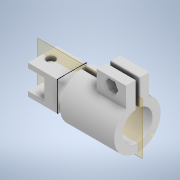
# Autodesk Inventor part: Arm connection
Saved by Autodesk Inventor 2021 (Build 250183000, 183)
## iProperties
Created: 2021-04-09
Part Number: Arm connection
Material: Generic
Document SubType Name: Modeling
Designer: Olivi
Density: 1 g/cm^3
Appearance: Default
Author: Olivi
Autodesk Inventor part; units mm, degrees
ref_plane "YZ Plane" through (0, 0, 0) normal (1, 0, 0) x (0, 1, 0)
sketch "Sketch1" plane through (0, 0, 0) normal (0, 0, 1) x (1, 0, 0)
  line L0 (0, 0) -> (0, 2.5)
  line L1 (0, 2.5) -> (8.5, 2.5)
  line L2 (8.5, 2.5) -> (8.5, 12.7)
  line L3 (8.5, 12.7) -> (0, 12.7)
  line L4 (0, 12.7) -> (0, 15.2)
  line L5 (0, 15.2) -> (15, 15.2)
  line L6 (15, 15.2) -> (15, 0)
  line L7 (15, 0) -> (0, 0)
  dimension "d0" = 2.5
  dimension "d1" = 8.5
  dimension "d2" = 10.2
  dimension "d3" = 2.5
  dimension "d4" = 15
  constraints: 16 end point, 6 perpendicular, 1 horizontal, 1 vertical
  measures "d0" distance of L0.start L0.end
  measures "d1" distance of L0.end L1.end
  measures "d2" distance of L1.end L2.end
  measures "d3" distance of L3.end L4.end
  measures "d4" distance of L4.end L5.end
extrude "Extrusion1" add sketch "Sketch1" along normal blind 15
ref_plane "Work Plane1" through (18, 0, 0) normal (1, 0, 0) x (0, 0, -1)
sketch "Sketch3" plane through (15, 0, 0) normal (1, 0, 0) x (0, 0, -1)
  line L0 (0, 15.2) -> (-15, 15.2) projected
  line L1 (-15, 15.2) -> (0, 15.2)
  line L2 (0, 0) -> (-15, 0) projected
  line L3 (0, 15.2) -> (0, 0)
  line L4 (-15, 2.5) -> (-15, 0) projected
  line L5 (0, 0) -> (-15, 0)
  line L6 (-15, 15.2) -> (-15, 12.7) projected
  line L7 (-15, 0) -> (-15, 15.2)
  constraints: 8 end point, 3 perpendicular, 1 horizontal
sketch "Sketch4" plane through (18, 0, 0) normal (1, 0, 0) x (0, 0, -1)
  circle A0 centre (-7.5, 7.7) radius 9
  line L0 (0, 15.2) -> (-15, 15.2) projected
  line L1 (-15, 0) -> (-15, 15.2) projected
  point P0 (0, 0)
  dimension "d10" = 18
  dimension "d11" = 7.5
  dimension "d12" = 7.5
  constraints: 1 centre point
  measures "d10" diameter of A0
  measures "d11" distance from line of L0 A0.centre
  measures "d12" distance from line of L1 A0.centre
ref_plane "Work Plane2" through (21, 7.7, 7.5) normal (1, 0, 0) x (0, 0, -1)
sketch "Sketch5" plane through (21, 7.7, 7.5) normal (1, 0, 0) x (0, 0, -1)
  circle A0 centre (0, 0) radius 12
  point P0 (7.5, -7.7)
  dimension "d18" = 24
  constraints: 1 centre point
  measures "d18" diameter of A0
sketch "Sketch4 outline for Loft2" plane through (18, 0, 0) normal (1, 0, 0) x (0, 0, -1)
  circle A0 centre (-7.5, 7.7) radius 9
sketch "Sketch5 outline for Loft2" plane through (21, 7.7, 7.5) normal (1, 0, 0) x (0, 0, -1)
  circle A0 centre (0, 0) radius 12
loft "Loft2" add profiles "Sketch4 outline for Loft2", "Sketch5 outline for Loft2" section 1 edges at (15, 7.6, 0) (15, 15.2, 7.5) (15, 7.6, 15) (15, 0, 7.5)
sketch "Sketch6" plane through (21, 7.7, 7.5) normal (1, 0, 0) x (0, 0, -1)
  circle A0 centre (0, 0) radius 7.75
  circle A1 centre (0, 0) radius 12
  point P0 (7.5, -7.7)
  dimension "d25" = 15.5
  constraints: 2 centre point, 1 coincident
  measures "d25" diameter of A0
extrude "Extrusion2" add sketch "Sketch6" along normal blind 28
ref_plane "Work Plane3" through (0, 0, 7.5) normal (0, 0, 1) x (1, 0, 0)
sketch "Sketch7" plane through (0, 0, 7.5) normal (0, 0, 1) x (1, 0, 0)
  line L0 (21, 19.7) -> (49, 19.7)
  line L1 (49, 19.7) -> (21, 19.7)
  line L2 (21, 16.241288) -> (21, -0.841288)
  line L3 (21, 15.217594) -> (49, 15.217594)
  line L4 (49, -4.3) -> (49, 19.7)
  line L5 (49, 15.217594) -> (49, 19.7)
  line L6 (21, 19.7) -> (21, 16.241288)
  line L7 (21, 19.7) -> (21, 15.217594)
  point P0 (0, 0)
  constraints: 8 end point, 3 point on line, 2 collinear, 1 perpendicular
extrude "Extrusion3" cut sketch "Sketch7" against normal mid plane 2
sketch "Sketch8" plane through (49, 7.7, 7.5) normal (1, 0, 0) x (0, 0, -1)
  point P0 (7.5, -7.7)
sketch "Sketch10" plane through (49, 7.7, 7.5) normal (1, 0, 0) x (0, 0, -1)
  arc A0 (-1, 11.958261) -> (-8.428903, 8.541288) centre (0, 0) ccw
  line L0 (-1, 11.958261) -> (-1, 20.958261)
  line L1 (-1, 20.958261) -> (-6, 20.958261)
  line L2 (-6, 20.958261) -> (-6, 10.392305)
  arc A1 (8.428903, 8.541288) -> (1, 11.958261) centre (0, 0) ccw
  line L3 (1, 11.958261) -> (1, 20.958261)
  line L4 (1, 20.958261) -> (6, 20.958261)
  line L5 (6, 20.958261) -> (6, 10.392305)
  arc A2 (-1, 11.958261) -> (-6, 10.392305) centre (0, 0) ccw
  line L6 (1, 7.685213) -> (1, 11.958261)
  arc A3 (6, 10.392305) -> (1, 11.958261) centre (0, 0) ccw
  point P0 (7.5, -7.7)
  dimension "d33" = 9
  dimension "d34" = 5
  dimension "d35" = 5
  constraints: 12 end point, 6 point on circle, 3 perpendicular, 2 centre point, 2 point on line, 1 concentric, 1 parallel, 1 vertical
  measures "d33" distance of L0.start L0.end
  measures "d34" distance of L0.end L1.end
  measures "d35" distance of L3.end L4.end
extrude "Extrusion4" add sketch "Sketch10" against normal blind 15
sketch "Sketch11" plane through (49, 18.092305, 1.5) normal (0, 0, -1) x (-1, 0, 0)
  circle A0 centre (7.5, 6.35) radius 1.75
  point P0 (49, -18.092305)
  dimension "d38" = 3.5
  constraints: 1 centre point
  measures "d38" diameter of A0
extrude "Extrusion5" cut sketch "Sketch11" against normal through all
sketch "Sketch12" plane through (49, 18.092305, 1.5) normal (0, 0, -1) x (-1, 0, 0)
  circle A0 centre (7.5, 6.35) radius 1.75 projected
  circle A1 centre (7.5, 6.35) radius 3
  point P0 (49, -18.092305)
  dimension "d41" = 6
  constraints: 1 centre point, 1 coincident
  measures "d41" diameter of A1
extrude "Extrusion6" cut sketch "Sketch12" against normal blind 2.5 contours A0 | A1
sketch "Sketch13" plane through (0, 0, 8.5) normal (0, 0, -1) x (-1, 0, 0)
  point P0 (0, 0)
sketch "Sketch14" plane through (49, 18.092305, 13.5) normal (0, 0, 1) x (1, 0, 0)
  circle A0 centre (-7.5, 6.35) radius 1.75
  line L0 (-3.920428, 6.35) -> (-5.710214, 3.25)
  line L1 (-5.710214, 3.25) -> (-9.289786, 3.25)
  line L2 (-9.289786, 3.25) -> (-11.079572, 6.35)
  line L3 (-11.079572, 6.35) -> (-9.289786, 9.45)
  line L4 (-9.289786, 9.45) -> (-5.710214, 9.45)
  line L5 (-5.710214, 9.45) -> (-3.920428, 6.35)
  point P0 (-49, -18.092305)
  dimension "d44" = 6.2
  constraints: 12 end point, 1 coincident, 13 other
  measures "d44" distance between parallel lines of L1 L4
extrude "Extrusion7" cut sketch "Sketch14" against normal blind 2.5
sketch "Sketch15" plane through (0, 2.5, 0) normal (0, 1, 0) x (1, 0, 0)
  circle A0 centre (4.3, -7.5) radius 2.25
  line L0 (8.5, 0) -> (8.5, -15) projected
  point P0 (0, 0)
  dimension "d47" = 4.5
  dimension "d48" = 4.2
  constraints: 1 centre point
  measures "d47" diameter of A0
  measures "d48" distance from line of L0 A0.centre
extrude "Extrusion8" cut sketch "Sketch15" along normal through all both and the other way through all
body "Solid1"
